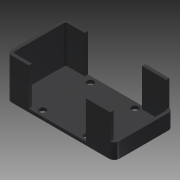
# Autodesk Inventor part: Batterie
Saved by Autodesk Inventor 2014 SP2 (Build 180246200, 246)
## iProperties
Created: 2015-03-18
Part Number: Batterie
Material: Plastique ABS
Document SubType Name: Modeling
Designer: sd
Mass: 34.3209 g
Surface Area: 65.7779 cm^2
Volume: 32.3782 cm^3
Density: 1.06 g/cm^3
Appearance: Lisse - Blanc
Author: sd
Autodesk Inventor part; units mm, degrees
ref_plane "YZ Plane" through (0, 0, 0) normal (1, 0, 0) x (0, 1, 0)
ref_plane "XZ Plane" through (0, 0, 0) normal (0, 1, 0) x (-1, 0, 0)
ref_plane "XY Plane" through (0, 0, 0) normal (0, 0, 1) x (1, 0, 0)
sketch "Esquisse1" plane through (0, 0, 0) normal (0, 1, 0) x (-1, 0, 0)
  line L0 (-26.924, -14.7955) -> (26.924, -14.7955)
  line L1 (26.924, -14.7955) -> (26.924, 14.7955)
  line L2 (26.924, 14.7955) -> (-26.924, 14.7955)
  line L3 (-26.924, 14.7955) -> (-26.924, -14.7955)
  point P0 (0, 0)
  dimension "d0" = 29.591
  dimension "d1" = 53.848
  dimension "d2" = 26.924
  dimension "d3" = 14.7955
  constraints: 8 end point, 2 parallel, 1 horizontal, 1 perpendicular
  measures "d0" distance of L2.end L0.start
  measures "d1" distance of L1.end L2.end
  measures "d2" horizontal distance of point (0, 0) L2.end
  measures "d3" vertical distance of point (0, 0) L2.end
extrude "Extrusion1" add sketch "Esquisse1" along normal blind 20.32
fillet "Congé1" radius 2.54 4 edges at (-26.924, 10.16, 14.7955) (26.924, 10.16, 14.7955) (26.924, 10.16, -14.7955) (-26.924, 10.16, -14.7955)
shell "Coque1" thickness 1.5875 removed faces 1 at (-8.128, 20.32, -4.9318)
sketch "Esquisse3" plane through (0, 20.32, 0) normal (0, 1, 0) x (1, 0, 0)
  line L0 (-26.924, 12.2555) -> (-26.924, -12.2555) projected
  line L1 (-24.384, -14.7955) -> (24.384, -14.7955) projected
  line L2 (-15.8115, 11.1125) -> (12.7635, 11.1125)
  line L3 (12.7635, 11.1125) -> (12.7635, 17.4625)
  line L4 (12.7635, 17.4625) -> (-15.8115, 17.4625)
  line L5 (-15.8115, 17.4625) -> (-15.8115, 11.1125)
  line L6 (-15.8115, -11.1125) -> (12.7635, -11.1125)
  line L7 (12.7635, -11.1125) -> (12.7635, -17.4625)
  line L8 (12.7635, -17.4625) -> (-15.8115, -17.4625)
  line L9 (-15.8115, -17.4625) -> (-15.8115, -11.1125)
  point P0 (0, 0)
  dimension "d8" = 28.575
  dimension "d9" = 28.575
  dimension "d10" = 11.1125
  dimension "d11" = 11.1125
  dimension "d12" = 6.35
  dimension "d13" = 6.35
  dimension "d14" = 22.225
  dimension "d15" = 2.667
  constraints: 16 end point, 4 parallel, 2 horizontal, 2 perpendicular
  measures "d8" distance of L3.end L4.end
  measures "d9" distance of L7.end L8.end
  measures "d10" distance between parallel lines of L0 L5
  measures "d11" distance between parallel lines of L0 L9
  measures "d12" distance of L2.end L3.end
  measures "d13" distance of L6.end L7.end
  measures "d14" distance from line of L2.end L6
  measures "d15" distance from line of L1 L7.end
extrude "Extrusion2" cut sketch "Esquisse3" against normal blind 18.7325
sketch "Esquisse4" plane through (0, 20.32, 0) normal (0, 1, 0) x (1, 0, 0)
  line L0 (24.8732, 15.6385) -> (27.4132, 15.6385)
  line L1 (27.4132, 15.6385) -> (27.4132, -16.1115)
  line L2 (27.4132, -16.1115) -> (24.8732, -16.1115)
  line L3 (24.8732, -16.1115) -> (24.8732, 15.6385)
  point P0 (0, 0)
  dimension "d18" = 31.75
  dimension "d19" = 2.54
  constraints: 8 end point, 2 parallel, 1 horizontal, 1 perpendicular
  measures "d18" distance of L0.end L1.end
  measures "d19" distance of L0.start L0.end
extrude "Extrusion3" cut sketch "Esquisse4" against normal blind 12.7
sketch "Esquisse5" plane through (25.3365, 1.5875, 12.2555) normal (0, 1, 0) x (1, 0, 0)
  line L0 (-50.673, 24.511) -> (-50.673, 0) projected
  line L1 (-12.573, -2.54) -> (-41.148, -2.54) projected
  circle A0 centre (-37.0205, 24.1808) radius 1.651
  circle A1 centre (-14.7955, 24.1808) radius 1.651
  circle A2 centre (-14.7955, 0.3556) radius 1.651
  circle A3 centre (-37.0205, 0.3556) radius 1.651
  circle A4 centre (-25.3365, 12.2555) radius 1.6
  line L2 (-49.7205, -2.54) -> (-41.148, -2.54) projected
  dimension "d22" = 3.302
  dimension "d23" = 3.302
  dimension "d24" = 3.302
  dimension "d25" = 3.302
  dimension "d26" = 3.2
  dimension "d27" = 23.8252
  dimension "d28" = 23.8252
  dimension "d29" = 22.225
  dimension "d30" = 22.225
  dimension "d31" = 2.8956
  dimension "d32" = 13.6525
  dimension "d33" = 2.8956
  dimension "d34" = 13.6525
  constraints: 5 centre point, 1 coincident
  measures "d22" diameter of A0
  measures "d23" diameter of A1
  measures "d24" diameter of A2
  measures "d25" diameter of A3
  measures "d26" diameter of A4
  measures "d27" distance of A2.centre A1.centre
  measures "d28" distance of A3.centre A0.centre
  measures "d29" distance of A2.centre A3.centre
  measures "d30" distance of A1.centre A0.centre
  measures "d31" distance from line of L2 A3.centre
  measures "d32" distance from line of L0 A3.centre
  measures "d33" distance from line of L1 A2.centre
  measures "d34" distance from line of L0 A0.centre
extrude "Extrusion4" cut sketch "Esquisse5" against normal through all
equation "\"d2\" = 0.5 * d1"
equation "\"d3\" = 0.5 * d0"
equation "\"d9\" = d8"
equation "\"d11\" = d10"
equation "\"d23\" = d22"
equation "\"d24\" = d22"
equation "\"d25\" = d22"
equation "\"d28\" = d27"
equation "\"d30\" = d29"
equation "\"d33\" = d31"
equation "\"d34\" = d32"
